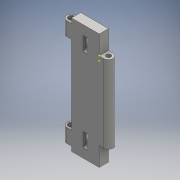
# Autodesk Inventor part: tracks
Saved by Autodesk Inventor 2016 (Build 200138000, 138)
## iProperties
Created: 2016-04-17
Part Number: tracks
Material: Generic
Document SubType Name: Modeling
Designer: Henrik Samuelsson
Density: 1 g/cm^3
Appearance: Default
Author: Henrik Samuelsson
Autodesk Inventor part; units mm, degrees
ref_plane "YZ Plane" through (0, 0, 0) normal (1, 0, 0) x (0, 1, 0)
ref_plane "XZ Plane" through (0, 0, 0) normal (0, 1, 0) x (-1, 0, 0)
ref_plane "XY Plane" through (0, 0, 0) normal (0, 0, 1) x (1, 0, 0)
sketch "Sketch1" plane through (0, 0, 0) normal (0, 1, 0) x (-1, 0, 0)
  line L0 (0, 0) -> (0, -8.2)
  line L1 (0, -8.2) -> (-4, -8.2)
  line L2 (-4, -8.2) -> (-4, -41.8)
  line L3 (-4, -41.8) -> (0, -41.8)
  line L4 (0, -41.8) -> (0, -50)
  line L5 (0, -50) -> (12, -50)
  line L6 (12, -50) -> (12, -48)
  line L7 (12, -48) -> (16, -48)
  line L8 (16, -48) -> (16, -42)
  line L9 (16, -42) -> (12, -42)
  line L10 (12, -42) -> (12, -8)
  line L11 (12, -8) -> (16, -8)
  line L12 (16, -8) -> (16, -2)
  line L13 (16, -2) -> (12, -2)
  line L14 (12, -2) -> (12, 0)
  line L15 (12, 0) -> (0, 0)
  line L16 (11, -4) -> (1, -4)
  line L17 (1, -4) -> (1, -10)
  line L18 (1, -10) -> (11, -10)
  line L19 (11, -10) -> (11, -4)
  line L20 (11, -40) -> (1, -40)
  line L21 (1, -40) -> (1, -46)
  line L22 (1, -46) -> (11, -46)
  line L23 (11, -46) -> (11, -40)
  dimension "d0" = 20
  dimension "d1" = 50
  dimension "d2" = 8.2
  dimension "d3" = 8.2
  dimension "d4" = 2
  dimension "d5" = 2
  dimension "d6" = 6
  dimension "d7" = 6
  dimension "d8" = 4
  dimension "d9" = 4
  dimension "d10" = 4
  dimension "d11" = 4
  dimension "d12" = 4
  dimension "d13" = 10
  dimension "d14" = 6
  dimension "d15" = 5
  dimension "d16" = 4
  dimension "d17" = 10
  dimension "d18" = 6
  dimension "d19" = 4
  constraints: 48 end point, 16 perpendicular, 4 parallel, 3 point on line, 2 horizontal, 1 vertical
  measures "d0" distance between parallel lines of L2 L12
  measures "d1" distance between parallel lines of L5 L15
  measures "d2" distance of L0.end L0.start
  measures "d3" distance of L4.end L3.end
  measures "d4" distance of L13.end L14.end
  measures "d5" distance of L5.end L6.end
  measures "d6" distance of L12.end L11.end
  measures "d7" distance of L7.end L8.end
  measures "d8" distance of L0.end L1.end
  measures "d9" distance of L13.end L12.end
  measures "d10" distance from line of L6 L7.end
  measures "d11" distance of L9.end L8.end
  measures "d12" distance from line of L10 L11.end
  measures "d13" distance of L17.end L18.end
  measures "d14" distance of L17.end L16.end
  measures "d15" distance from line of L2 L17.end
  measures "d16" distance from line of L15 L16.start
  measures "d17" distance of L21.end L22.end
  measures "d18" distance of L21.end L20.end
  measures "d19" distance between parallel lines of L5 L22
extrude "Extrusion1" add sketch "Sketch1" along normal blind 4
sketch "Sketch2" plane through (-11, 0, -10) normal (0, 0, 1) x (1, 0, 0)
  point P0 (11, 0)
ref_plane "Work Plane1" through (-6, 4, -10) normal (0, 0, 1) x (1, 0, 0)
sketch "Sketch4" plane through (-6, 4, -10) normal (0, 0, 1) x (1, 0, 0)
  line L0 (-5, -4) -> (5, -4) projected
  line L1 (5, -4) -> (-5, -4) projected
  line L2 (-5, -4) -> (5, -4) projected
  line L3 (5, -4) -> (-5, -4) projected
  line L4 (-6, -4) -> (6, -4) projected
  line L5 (-10, -4) -> (-6, -4) projected
  line L6 (-6, -4) -> (-10, -4) projected
  line L7 (-10, -4) -> (-6, -4) projected
  line L8 (-6, -4) -> (-10, -4) projected
  line L9 (6, -4) -> (-6, -4) projected
  line L10 (10, -4) -> (6, -4) projected
  line L11 (6, -4) -> (10, -4) projected
  line L12 (-5, 0) -> (5, 0) projected
  line L13 (5, 0) -> (-5, 0) projected
  line L14 (-5, 0) -> (5, 0) projected
  line L15 (5, 0) -> (-5, 0) projected
  line L16 (6, 0) -> (10, 0) projected
  line L17 (10, 0) -> (6, 0) projected
  line L18 (6, 0) -> (-6, 0) projected
  line L19 (-6, 0) -> (-10, 0) projected
  line L20 (-10, 0) -> (-6, 0) projected
  line L21 (-6, 0) -> (-10, 0) projected
  line L22 (-10, 0) -> (-6, 0) projected
  line L23 (-6, 0) -> (6, 0) projected
  line L24 (5, -4) -> (5, 0) projected
  line L25 (-5, -4) -> (-5, 0) projected
  line L26 (6, -4) -> (-6, -4) projected
  arc A0 (-1, -4) -> (-5, 0) centre (-5, -4) ccw
  line L27 (-5, -4) -> (-5, 0) construction
  line L28 (-5, -4) -> (-1, -4) construction
  line L29 (5, -4) -> (5, 0) projected
  arc A1 (5, 0) -> (1, -4) centre (5, -4) ccw
  line L30 (5, -4) -> (5, 0) construction
  line L31 (5, -4) -> (9, -4) construction
  line L32 (-5, 0) -> (-5, -4)
  line L33 (-5, -4.2291) -> (-1, -4.2291)
  line L34 (1, -4) -> (5, -4)
  line L35 (5, 0) -> (5, -4)
  line L36 (6, 0) -> (-6, 0) projected
  line L37 (-5, -4) -> (-1, -4)
  dimension "d25" = 4
  dimension "d26" = 90
  dimension "d27" = 4
  dimension "d28" = 90
  constraints: 18 end point, 4 point on circle, 3 collinear, 2 centre point, 2 coincident, 1 horizontal, 1 parallel, 1 perpendicular, 1 point on line, 1 vertical, 3 other
  measures "d25" radius of A0
  measures "d26" angle of L28 L27
  measures "d27" radius of A1
  measures "d28" angle of L31 L30
extrude "Extrusion2" add sketch "Sketch4" along normal blind 6 contours L25 A0 L0 | A1 L24 L0
sketch "Sketch5" plane through (-1, 0, -40) normal (0, 0, -1) x (-1, 0, 0)
  line L0 (11, 0) -> (-1, 0) projected
  arc A0 (4, 0) -> (0, 4) centre (0, 0) ccw
  arc A1 (10, 4) -> (6, 0) centre (10, 0) ccw
  line L1 (0, 4) -> (0, 0)
  line L2 (0, 0) -> (4, 0)
  line L3 (6, 0) -> (10, 0)
  line L4 (10, 4) -> (10, 0)
  line L5 (11, 4) -> (-1, 4) projected
  point P0 (0, 4)
  constraints: 8 end point, 4 point on circle, 2 centre point, 2 collinear, 2 point on line, 1 perpendicular, 1 vertical
extrude "Extrusion3" add sketch "Sketch5" along normal blind 6 contours L0 A1 L4 | L0 L1 A0
sketch "Sketch6" plane through (-12, 0, -48) normal (0, 0, -1) x (-1, 0, 0)
  circle A0 centre (2, 2) radius 1.3
  line L0 (0, 0) -> (4, 0) projected
  line L1 (4, 0) -> (4, 4) projected
  line L2 (0, 4) -> (4, 4) projected
  line L3 (0, 0) -> (0, 4) projected
  point P0 (-12, 0)
  dimension "d33" = 2.6
  dimension "d34" = 2
  dimension "d35" = 2
  constraints: 1 centre point
  measures "d33" diameter of A0
  measures "d34" distance from line of L0 A0.centre
  measures "d35" distance from line of L1 A0.centre
extrude "Extrusion4" cut sketch "Sketch6" against normal through all contours A0
sketch "Sketch7" plane through (4, 0, -41.8) normal (0, 0, -1) x (-1, 0, 0)
  circle A0 centre (2, 2) radius 1
  line L0 (0, 4) -> (4, 4) projected
  line L1 (0, 0) -> (0, 4) projected
  point P0 (4, 0)
  dimension "d38" = 2
  dimension "d39" = 2
  dimension "d40" = 2
  constraints: 1 centre point
  measures "d38" diameter of A0
  measures "d39" distance from line of L1 A0.centre
  measures "d40" distance from line of L0 A0.centre
extrude "Extrusion5" cut sketch "Sketch7" against normal through all
sketch "Sketch8" plane through (-12, 0, -8) normal (0, 0, -1) x (-1, 0, 0)
  point P0 (-12, 0)
fillet "Fillet1" radius 2 2 edges at (-16, 4, -5) (-16, 0, -5)
fillet "Fillet2" radius 2 1 edges at (-16, 0, -45)
fillet "Fillet3" radius 2 1 edges at (-16, 4, -45)
fillet "Fillet4" radius 2 2 edges at (4, 4, -25) (4, 0, -25)
sketch "Sketch11" plane through (0, 0, -8.2) normal (0, 0, 1) x (1, 0, 0)
  point P0 (0, 0)
body "Solid1"
